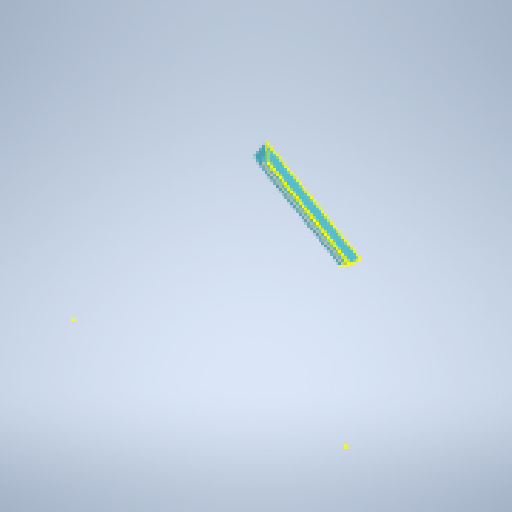
# Autodesk Inventor part: Perfil_V3
Saved by Autodesk Inventor 2024.2 (Build 282272000, 272)
## iProperties
Created: 2023-08-17
Part Number: Perfil_V3
Material: Genérico
Document SubType Name: Modeling
Designer: sergi
Density: 1 g/cm^3
Appearance: Valor por defecto
Author: sergi
Autodesk Inventor part; units mm, degrees
ref_plane "YZ Plane" through (0, 0, 0) normal (1, 0, 0) x (0, 1, 0)
ref_plane "XZ Plane" through (0, 0, 0) normal (0, 1, 0) x (-1, 0, 0)
ref_plane "XY Plane" through (0, 0, 0) normal (0, 0, 1) x (1, 0, 0)
sketch "Boceto2" plane through (0, 0, 0) normal (0, 1, 0) x (-1, 0, 0)
  line L0 (0, -100.3768) -> (-95.464, -31.0181)
  line L1 (-95.464, -31.0181) -> (-59, 81.2065)
  line L2 (-59, 81.2065) -> (59, 81.2065)
  line L3 (59, 81.2065) -> (95.464, -31.0181)
  line L4 (95.464, -31.0181) -> (0, -100.3768)
  line L5 (0, 0) -> (162.4131, 0) construction
  line L6 (162.4131, 0) -> (162.4131, 162.4131) construction
  line L7 (162.4131, 162.4131) -> (0, 162.4131) construction
  line L8 (0, 162.4131) -> (0, 0) construction
  line L9 (162.4131, 162.4131) -> (0, 81.2065) construction
  dimension "Lado" = 118
  dimension "d1" = 26.565
  dimension "d2" = 262.7899
  constraints: 20 end point, 2 horizontal, 2 midpoint, 2 parallel, 2 perpendicular, 1 coincident, 11 other
  measures "Lado" distance of L1.end L2.end
  measures "d1" angle of L2 L9
  measures "d2" distance from line of L0.start L7
extrude "Extrusión1" add sketch "Boceto2" along normal blind 262.7899 draft 26.565
sketch "Boceto3" plane through (0, 262.7899, 0) normal (0, 1, 0) x (1, 0, 0)
  line L0 (0, -100.3768) -> (-95.464, -31.0181)
  line L1 (-95.464, -31.0181) -> (-59, 81.2065)
  line L2 (-59, 81.2065) -> (59, 81.2065)
  line L3 (59, 81.2065) -> (95.464, -31.0181)
  line L4 (95.464, -31.0181) -> (0, -100.3768)
  point P0 (0, 0)
  point P1 (0, 0)
  dimension "d5" = 118
  constraints: 10 end point, 1 coincident, 1 horizontal, 11 other
  measures "d5" distance of L1.end L2.end
extrude "Extrusión2" cut sketch "Boceto3" against normal blind 262.7899 draft 26.565 keep common part
sketch "Boceto4" plane through (-95.464, 262.7899, 31.0181) normal (-0.5257311, 0.4472136, 0.7236068) x (0.809017, 0, 0.5877853)
  line L0 (-36.464, -112.2247) -> (59, -181.5833) projected
  line L1 (59, -181.5833) -> (154.464, -112.2247) projected
  line L2 (118, 0) -> (154.464, -112.2247) projected
  line L3 (118, 0) -> (0, 0) projected
  line L4 (0, 0) -> (-36.464, -112.2247) projected
  line L5 (59, -167.9866) -> (-23.5327, -108.023)
  line L6 (-23.5327, -108.023) -> (7.992, -11)
  line L7 (7.992, -11) -> (110.008, -11)
  line L8 (110.008, -11) -> (141.5327, -108.023)
  line L9 (141.5327, -108.023) -> (59, -167.9866)
  point P0 (59, -198.7297)
  dimension "Ancho_Marco" = 11
  constraints: 10 end point, 4 other
  measures "Ancho_Marco" distance between parallel lines of L0 L5
extrude "Extrusión3" cut sketch "Boceto4" against normal blind 162.7899 contours L5 L6 L7 L8 L9
sketch "Boceto5" plane through (-59, 0, 81.2065) normal (0, -0.4472136, 0.8944272) x (1, 0, 0)
  line L0 (-36.464, 112.2247) -> (59, 181.5833) projected
  line L1 (0, 0) -> (-36.464, 112.2247) projected
  line L2 (0, 0) -> (118, 0) projected
  line L3 (118, 0) -> (154.464, 112.2247) projected
  line L4 (59, 181.5833) -> (154.464, 112.2247) projected
  line L5 (-23.5327, 108.023) -> (59, 167.9866)
  line L6 (59, 167.9866) -> (141.5327, 108.023)
  line L7 (141.5327, 108.023) -> (110.008, 11)
  line L8 (110.008, 11) -> (7.992, 11)
  line L9 (7.992, 11) -> (-23.5327, 108.023)
  point P0 (59, -36.3167)
  dimension "d11" = 11
  constraints: 10 end point, 4 other
  measures "d11" distance between parallel lines of L1 L9
sketch "Boceto6" plane through (-95.464, 0, -31.0181) normal (-0.8506508, -0.4472136, 0.2763932) x (0.309017, 0, 0.9510565)
  line L0 (-36.464, 112.2247) -> (59, 181.5833) projected
  line L1 (0, 0) -> (-36.464, 112.2247) projected
  line L2 (0, 0) -> (118, 0) projected
  line L3 (118, 0) -> (154.464, 112.2247) projected
  line L4 (59, 181.5833) -> (154.464, 112.2247) projected
  line L5 (-23.5327, 108.023) -> (59, 167.9866)
  line L6 (59, 167.9866) -> (141.5327, 108.023)
  line L7 (141.5327, 108.023) -> (110.008, 11)
  line L8 (110.008, 11) -> (7.992, 11)
  line L9 (7.992, 11) -> (-23.5327, 108.023)
  point P0 (59, -36.3167)
  dimension "d12" = 11
  constraints: 10 end point, 4 other
  measures "d12" distance between parallel lines of L1 L9
sketch "Boceto7" plane through (-59, 262.7899, -81.2065) normal (-0.8506508, 0.4472136, -0.2763932) x (-0.309017, 0, 0.9510565)
  line L0 (-36.464, -112.2247) -> (59, -181.5833) projected
  line L1 (59, -181.5833) -> (154.464, -112.2247) projected
  line L2 (118, 0) -> (154.464, -112.2247) projected
  line L3 (118, 0) -> (0, 0) projected
  line L4 (0, 0) -> (-36.464, -112.2247) projected
  line L5 (59, -167.9866) -> (-23.5327, -108.023)
  line L6 (-23.5327, -108.023) -> (7.992, -11)
  line L7 (7.992, -11) -> (110.008, -11)
  line L8 (110.008, -11) -> (141.5327, -108.023)
  line L9 (141.5327, -108.023) -> (59, -167.9866)
  point P0 (59, -198.7297)
  dimension "d13" = 11
  constraints: 10 end point, 4 other
  measures "d13" distance between parallel lines of L0 L5
sketch "Boceto8" plane through (0, 262.7899, 0) normal (0, 1, 0) x (1, 0, 0)
  line L0 (-59, 81.2065) -> (59, 81.2065) projected
  line L1 (-95.464, -31.0181) -> (-59, 81.2065) projected
  line L2 (0, -100.3768) -> (-95.464, -31.0181) projected
  line L3 (95.464, -31.0181) -> (0, -100.3768) projected
  line L4 (59, 81.2065) -> (95.464, -31.0181) projected
  line L5 (-82.5327, -26.8165) -> (-51.008, 70.2065)
  line L6 (-51.008, 70.2065) -> (51.008, 70.2065)
  line L7 (51.008, 70.2065) -> (82.5327, -26.8165)
  line L8 (82.5327, -26.8165) -> (0, -86.78)
  line L9 (0, -86.78) -> (-82.5327, -26.8165)
  point P0 (0, 0)
  dimension "d14" = 11
  constraints: 10 end point, 4 other
  measures "d14" distance between parallel lines of L2 L9
sketch "Boceto9" plane through (0, 262.7899, 100.3768) normal (0.5257311, 0.4472136, 0.7236068) x (0.809017, 0, -0.5877853)
  line L0 (-36.464, -112.2247) -> (59, -181.5833) projected
  line L1 (59, -181.5833) -> (154.464, -112.2247) projected
  line L2 (118, 0) -> (154.464, -112.2247) projected
  line L3 (118, 0) -> (0, 0) projected
  line L4 (0, 0) -> (-36.464, -112.2247) projected
  line L5 (7.992, -11) -> (110.008, -11)
  line L6 (110.008, -11) -> (141.5327, -108.023)
  line L7 (141.5327, -108.023) -> (59, -167.9866)
  line L8 (59, -167.9866) -> (-23.5327, -108.023)
  line L9 (-23.5327, -108.023) -> (7.992, -11)
  point P0 (59, -198.7297)
  dimension "d15" = 11
  constraints: 10 end point, 4 other
  measures "d15" distance between parallel lines of L3 L5
extrude "Extrusión4" cut sketch "Boceto7" against normal blind 162.7899 contours L5 L6 L7 L8 L9
extrude "Extrusión5" cut sketch "Boceto8" against normal blind 162.7899 contours L5 L6 L7 L8 L9
extrude "Extrusión6" cut sketch "Boceto9" against normal blind 162.7899 contours L5 L6 L7 L8 L9
extrude "Extrusión7" cut sketch "Boceto5" against normal blind 162.7899 contours L5 L6 L7 L8 L9
extrude "Extrusión8" cut sketch "Boceto6" against normal blind 162.7899 contours L5 L6 L7 L8 L9
sketch "Boceto10" plane through (59, 0, 81.2065) normal (0.8506508, -0.4472136, 0.2763932) x (0.309017, 0, -0.9510565)
  line L0 (59, 181.5833) -> (154.464, 112.2247) projected
  line L1 (-36.464, 112.2247) -> (59, 181.5833) projected
  line L2 (0, 0) -> (-36.464, 112.2247) projected
  line L3 (0, 0) -> (118, 0) projected
  line L4 (118, 0) -> (154.464, 112.2247) projected
  line L5 (-23.5327, 108.023) -> (59, 167.9866)
  line L6 (59, 167.9866) -> (141.5327, 108.023)
  line L7 (141.5327, 108.023) -> (110.008, 11)
  line L8 (110.008, 11) -> (7.992, 11)
  line L9 (7.992, 11) -> (-23.5327, 108.023)
  point P0 (59, -36.3167)
  dimension "d26" = 11
  constraints: 10 end point, 4 other
  measures "d26" distance between parallel lines of L2 L9
sketch "Boceto11" plane through (0, 0, 0) normal (0, -1, 0) x (1, 0, 0)
  line L0 (-59, 81.2065) -> (59, 81.2065) projected
  line L1 (-82.5327, 26.8165) -> (0, 86.78) projected
  line L2 (-95.464, -31.0181) -> (-59, 81.2065) projected
  line L3 (0, -100.3768) -> (-95.464, -31.0181) projected
  line L4 (95.464, -31.0181) -> (0, -100.3768) projected
  line L5 (59, 81.2065) -> (95.464, -31.0181) projected
  line L6 (-59, 81.2065) -> (59, 81.2065) projected
  line L7 (-51.008, 70.2065) -> (-82.5327, -26.8165)
  line L8 (-82.5327, -26.8165) -> (0, -86.78)
  line L9 (0, -86.78) -> (82.5327, -26.8165)
  line L10 (82.5327, -26.8165) -> (51.008, 70.2065)
  line L11 (51.008, 70.2065) -> (-51.008, 70.2065)
  point P0 (0, 0)
  point P1 (-22.8115, 70.2065)
  point P2 (-59.7212, 43.39)
  dimension "d27" = 11
  constraints: 10 end point, 4 other
  measures "d27" distance between parallel lines of L2 L7
sketch "Boceto12" plane through (0, 0, -100.3768) normal (-0.5257311, -0.4472136, -0.7236068) x (-0.809017, 0, 0.5877853)
  line L0 (78.4833, 87.5371) -> (69.2036, 84.5219) projected
  line L1 (59, 181.5833) -> (154.464, 112.2247) projected
  line L2 (-36.464, 112.2247) -> (59, 181.5833) projected
  line L3 (0, 0) -> (-36.464, 112.2247) projected
  line L4 (0, 0) -> (118, 0) projected
  line L5 (118, 0) -> (154.464, 112.2247) projected
  line L6 (141.5327, 108.023) -> (59, 167.9866)
  line L7 (59, 167.9866) -> (-23.5327, 108.023)
  line L8 (-23.5327, 108.023) -> (7.992, 11)
  line L9 (7.992, 11) -> (110.008, 11)
  line L10 (110.008, 11) -> (141.5327, 108.023)
  point P0 (59, -36.3167)
  point P1 (59, 91.9353)
  point P2 (69, 94.9704)
  point P3 (69.2036, 84.5219)
  dimension "d28" = 11
  constraints: 10 end point, 5 other
  measures "d28" distance between parallel lines of L5 L10
sketch "Boceto13" plane through (59, 262.7899, -81.2065) normal (0, 0.4472136, -0.8944272) x (-1, 0, 0)
  line L0 (59, -181.5833) -> (154.464, -112.2247) projected
  line L1 (118, 0) -> (154.464, -112.2247) projected
  line L2 (118, 0) -> (0, 0) projected
  line L3 (0, 0) -> (-36.464, -112.2247) projected
  line L4 (-36.464, -112.2247) -> (59, -181.5833) projected
  line L5 (141.5327, -108.023) -> (59, -167.9866)
  line L6 (59, -167.9866) -> (-23.5327, -108.023)
  line L7 (-23.5327, -108.023) -> (7.992, -11)
  line L8 (7.992, -11) -> (110.008, -11)
  line L9 (110.008, -11) -> (141.5327, -108.023)
  point P0 (59, -198.7297)
  dimension "d29" = 11
  constraints: 10 end point, 4 other
  measures "d29" distance between parallel lines of L1 L9
sketch "Boceto14" plane through (95.464, 262.7899, 31.0181) normal (0.8506508, 0.4472136, -0.2763932) x (-0.309017, 0, -0.9510565)
  line L0 (59, -181.5833) -> (154.464, -112.2247) projected
  line L1 (118, 0) -> (154.464, -112.2247) projected
  line L2 (118, 0) -> (0, 0) projected
  line L3 (0, 0) -> (-36.464, -112.2247) projected
  line L4 (-36.464, -112.2247) -> (59, -181.5833) projected
  line L5 (141.5327, -108.023) -> (59, -167.9866)
  line L6 (59, -167.9866) -> (-23.5327, -108.023)
  line L7 (-23.5327, -108.023) -> (7.992, -11)
  line L8 (7.992, -11) -> (110.008, -11)
  line L9 (110.008, -11) -> (141.5327, -108.023)
  point P0 (59, -198.7297)
  dimension "d30" = 11
  constraints: 10 end point, 4 other
  measures "d30" distance between parallel lines of L1 L9
sketch "Boceto15" plane through (95.464, 0, -31.0181) normal (0.5257311, -0.4472136, -0.7236068) x (-0.809017, 0, -0.5877853)
  line L0 (59, 181.5833) -> (154.464, 112.2247) projected
  line L1 (-36.464, 112.2247) -> (59, 181.5833) projected
  line L2 (0, 0) -> (-36.464, 112.2247) projected
  line L3 (0, 0) -> (118, 0) projected
  line L4 (118, 0) -> (154.464, 112.2247) projected
  line L5 (141.5327, 108.023) -> (59, 167.9866)
  line L6 (59, 167.9866) -> (-23.5327, 108.023)
  line L7 (-23.5327, 108.023) -> (7.992, 11)
  line L8 (7.992, 11) -> (110.008, 11)
  line L9 (110.008, 11) -> (141.5327, 108.023)
  point P0 (59, -36.3167)
  dimension "d31" = 11
  constraints: 10 end point, 4 other
  measures "d31" distance between parallel lines of L0 L5
extrude "Extrusión9" cut sketch "Boceto13" against normal blind 162.7899 contours L5 L6 L7 L8 L9
extrude "Extrusión10" cut sketch "Boceto15" against normal blind 162.7899 contours L9 L8 L7 L6 L5
extrude "Extrusión11" cut sketch "Boceto14" against normal blind 162.7899 contours L5 L6 L7 L8 L9
extrude "Extrusión12" cut sketch "Boceto12" against normal blind 162.7899 contours L10 L9 L8 L7 L6
extrude "Extrusión13" cut sketch "Boceto11" against normal blind 162.7899 contours L11 L10 L9 L8 L7 L1 | L1 L7 L11
extrude "Extrusión14" cut sketch "Boceto10" against normal blind 162.7899 contours L5 L6 L7 L8 L9
ref_plane "Plano de trabajo1" through (93.3374, 261.6718, 31.7091) normal (0.8506508, 0.4472136, -0.2763932) x (-0.309017, 0, -0.9510565)
sketch "Boceto17" plane through (93.3374, 261.6718, 31.7091) normal (0.8506508, 0.4472136, -0.2763932) x (-0.309017, 0, -0.9510565)
  line L0 (-23.5327, -108.023) -> (7.992, -11) projected
  line L1 (7.992, -11) -> (110.008, -11) projected
  line L2 (110.008, -11) -> (141.5327, -108.023) projected
  line L3 (141.5327, -108.023) -> (59, -167.9866) projected
  line L4 (59, -167.9866) -> (-23.5327, -108.023) projected
  line L5 (59, -181.5833) -> (154.464, -112.2247) projected
  line L6 (118, 0) -> (154.464, -112.2247) projected
  line L7 (118, 0) -> (0, 0) projected
  line L8 (0, 0) -> (-36.464, -112.2247) projected
  line L9 (-36.464, -112.2247) -> (59, -181.5833) projected
  line L10 (59, -172.9309) -> (146.235, -109.5509)
  line L11 (146.235, -109.5509) -> (112.9142, -7)
  line L12 (112.9142, -7) -> (5.0858, -7)
  line L13 (5.0858, -7) -> (-28.235, -109.5509)
  line L14 (-28.235, -109.5509) -> (59, -172.9309)
  point P0 (59, -198.7297)
  dimension "d48" = 4
  constraints: 10 end point, 4 other
  measures "d48" distance between parallel lines of L3 L10
extrude "Extrusión15" cut sketch "Boceto17" against normal blind 1.8 contours L14 L13 L12 L11 L10
ref_plane "Plano de trabajo4" through (61.2404, 249.7138, -72.2169) normal (0.5, 0.5257311, -0.688191) x (0.309017, -0.8506508, -0.4253254)
ref_plane "Plano de trabajo3" through (62.4904, 251.0281, -73.9374) normal (0.5, 0.5257311, -0.688191) x (0.309017, -0.8506508, -0.4253254)
ref_plane "Plano de trabajo5" through (97.6729, 166.1711, -118.5159) normal (0.5, -0.8506508, 0.1624598) x (-0.8506508, -0.4472136, 0.2763932)
ref_plane "Plano de trabajo6" through (82.5327, 166.1711, -129.5159) normal (-0.309017, -0.8506508, -0.4253254) x (0, -0.4472136, 0.8944272)
split "Dividir2" plane through (97.6729, 166.1711, -118.5159) removes the side toward (0.5, -0.8506508, 0.1624598)
split "Dividir3" plane through (82.5327, 166.1711, -129.5159) removes the side toward (-0.309017, -0.8506508, -0.4253254)
ref_plane "Plano de trabajo7" through (66.1482, 252.9512, -75.1259) normal (0, 0.5257311, 0.8506508) x (-0.8506508, -0.4472136, 0.2763932)
ref_plane "Plano de trabajo8" through (51.008, 252.9512, -86.1259) normal (-0.809017, 0.5257311, 0.2628656) x (0, -0.4472136, 0.8944272)
split "Dividir4" plane through (66.1482, 252.9512, -75.1259) removes the side toward (0, 0.5257311, 0.8506508)
split "Dividir5" plane through (51.008, 252.9512, -86.1259) removes the side toward (-0.809017, 0.5257311, 0.2628656)
split "Dividir6" plane through (61.2404, 249.7138, -72.2169) removes the side toward (-0.5, -0.5257311, 0.688191)
ref_plane "Plano de trabajo9" through (-14.2309, 126.771, 19.5872) normal (-0.809017, 0, -0.5877853) x (0.5773503, 0.1875925, -0.7946545)
mirror "Simetría1" about plane through (-14.2309, 126.771, 19.5872) normal (-0.809017, 0, -0.5877853) of "Extrusión15"
sketch "Boceto19" plane through (91.5151, 162.9338, -116.5151) normal (-0.5, -0.5257311, 0.688191) x (0.809017, 0, 0.5877853)
  line L0 (-5.5514, -3.431) -> (-11.1029, 0) projected
  line L1 (0, 0) -> (-5.5514, -3.431) projected
  line L2 (0, 102.0161) -> (0, 0) projected
  line L3 (-5.5514, 105.447) -> (0, 102.0161) projected
  line L4 (-11.1029, 102.0161) -> (-5.5514, 105.447) projected
  line L5 (-11.1029, 0) -> (-11.1029, 102.0161) projected
  point P0 (-5.5514, -60.7632)
  dimension "d54" = 11.1029
  dimension "d55" = 102.0161
  measures "d54" distance between parallel lines of L5 L2
  measures "d55" distance of L2.start L1.start
sketch "Boceto20" plane through (91.8062, 260.8668, 32.2066) normal (0.8506508, 0.4472136, -0.2763932) x (-0.309017, 0, -0.9510565)
  line L0 (112.9142, -7) -> (110.008, -11) projected
  line L1 (141.5327, -108.023) -> (110.008, -11) projected
  line L2 (141.5327, -108.023) -> (146.235, -109.5509) projected
  line L3 (112.9142, -7) -> (146.235, -109.5509) projected
  point P0 (59, -198.7297)
fillet "Empalme1" radius 1 4 edges at (79.7857, 208.444, -96.1305) (78.2511, 207.6372, -95.6319) (66.7704, 208.444, -105.5866) (66.7704, 207.6372, -103.9731)
sketch "Boceto21" plane through (95.464, 162.4131, -131.3949) normal (0, 0.4472136, -0.8944272) x (-0.9510565, 0.2763932, 0.1381966)
  line L0 (69.3587, 95.464) -> (0, 0) projected
  line L1 (73.5603, 82.5327) -> (69.3587, 95.464) projected
  line L2 (69.3587, 95.464) -> (0, 0) projected
  line L3 (0, 0) -> (13.5967, 0) projected
  line L4 (13.5967, 0) -> (73.5603, 82.5327) projected
  line L5 (13.5967, 0) -> (7.992, 11)
  line L6 (13.5967, 0) -> (25.9423, 0) construction
  point P0 (64.0601, -111.7712)
  dimension "d63" = 126
  dimension "d64" = 117
  constraints: 4 end point, 1 equal length, 1 horizontal, 1 point on line
  measures "d63" angle of L3 L4
  measures "d64" angle of L6 L5
sketch "Boceto22" plane through (97.6729, 166.1711, -118.5159) normal (0.8506508, 0.4472136, -0.2763932) x (-0.1624598, -0.2763932, -0.9472136)
  line L0 (-55.7619, 95.464) -> (-59.9635, 82.5327) projected
  line L1 (-59.9635, 82.5327) -> (0, 0) projected
  line L2 (0, 0) -> (13.5967, 0) projected
  line L3 (-55.7619, 95.464) -> (13.5967, 0) projected
  line L4 (-59.9635, 82.5327) -> (0, 0) projected
  line L5 (1.2361, 0) -> (-59.5816, 83.7083) projected
  point P0 (-50.4634, -111.7712)
  dimension "d65" = 11
  measures "d65" distance between parallel lines of L3 L4
sketch "Boceto23" plane through (93.2119, 162.8815, -122.0107) normal (0.5, -0.8506508, 0.1624598) x (0.8506508, 0.4472136, -0.2763932)
  ellipse E0 centre (-1, 3.7082) end of major axis (-1, 4.9443) minor radius 1 (0, 3.7082) -> (-1, 4.9443) ccw projected
  line L0 (-1, 4.9443) -> (-2.9389, 4.9443) projected
  line L1 (-2.9389, 4.9443) -> (-5.8575, -0.8928) projected
  line L2 (-5.8575, -0.8928) -> (4.3, -8.6525) projected
  line L3 (4.3, 4.9443) -> (4.3, -8.6525) projected
  line L4 (4.3, 4.9443) -> (2.8, 4.9443) projected
  ellipse E1 centre (2.8, 3.7082) end of major axis (2.8, 4.9443) minor radius 1 (2.8, 4.9443) -> (1.8, 3.7082) ccw projected
  line L5 (1.8, 0) -> (1.8, 3.7082) projected
  line L6 (1.8, 0) -> (0, 0) projected
  line L7 (0, 3.7082) -> (0, 0) projected
  line L8 (1.8, 0) -> (1.8, 4.9443)
  point P0 (-185.8565, 55.4077)
  dimension "d67" = 4.9443
  constraints: 2 end point, 2 point on line, 2 other
  measures "d67" distance of L5.start L8.end
ref_plane "Plano de trabajo2" through (59.2794, 271.8594, -65.6718) normal (0.5, 0.5257311, -0.688191) x (0.309017, -0.8506508, -0.4253254)
equation "\"d3\" = d2"
equation "\"d4\" = d1"
equation "\"d5\" = Lado"
equation "\"d6\" = d2"
equation "\"d7\" = d1"
equation "\"d11\" = Ancho_Marco"
equation "\"d12\" = Ancho_Marco"
equation "\"d13\" = Ancho_Marco"
equation "\"d14\" = Ancho_Marco"
equation "\"d15\" = Ancho_Marco"
equation "\"d26\" = Ancho_Marco"
equation "\"d27\" = Ancho_Marco"
equation "\"d28\" = Ancho_Marco"
equation "\"d29\" = Ancho_Marco"
equation "\"d30\" = Ancho_Marco"
equation "\"d31\" = Ancho_Marco"
